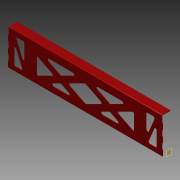
# Autodesk Inventor part: Front
Saved by Autodesk Inventor 2015 (Build 190159000, 159)
## iProperties
Created: 2014-01-06
Part Number: Front
Material: Aluminum 6061
Document SubType Name: Sheet Metal
Designer: Alex
Density: 2.71 g/cm^3
Sheet Metal Rule: Default
Appearance: Red
Author: Alex
Autodesk Inventor part; units mm, degrees
ref_plane "YZ Plane" through (0, 0, 0) normal (1, 0, 0) x (0, 1, 0)
ref_plane "XZ Plane" through (0, 0, 0) normal (0, 1, 0) x (-1, 0, 0)
ref_plane "XY Plane" through (0, 0, 0) normal (0, 0, 1) x (1, 0, 0)
sketch "Sketch1" plane through (0, 0, 0) normal (0, 0, 1) x (1, 0, 0)
  line L0 (-18.5351, 198.7023) -> (673.8689, 198.7023)
  line L1 (673.8689, 198.7023) -> (673.8689, -4.4977)
  line L2 (673.8689, -4.4977) -> (-18.5351, -4.4977)
  line L3 (-18.5351, -4.4977) -> (-18.5351, 198.7023)
  line L4 (-18.5351, 198.7023) -> (-15.9951, 198.7023)
  line L5 (-15.9951, 198.7023) -> (-15.9951, 173.3023)
  line L6 (-15.9951, 173.3023) -> (-18.5351, 173.3023)
  line L7 (-18.5351, 173.3023) -> (-18.5351, 198.7023)
  line L8 (-18.5351, -4.4977) -> (-15.9951, -4.4977)
  line L9 (-15.9951, -4.4977) -> (-15.9951, 20.9023)
  line L10 (-15.9951, 20.9023) -> (-18.5351, 20.9023)
  line L11 (-18.5351, 20.9023) -> (-18.5351, -4.4977)
  line L12 (-18.5351, 71.7023) -> (-15.9951, 71.7023)
  line L13 (-15.9951, 46.3023) -> (-18.5351, 46.3023)
  line L14 (-18.5351, 46.3023) -> (-18.5351, 71.7023)
  line L15 (-18.5351, 147.9023) -> (-15.9951, 147.9023)
  line L16 (-15.9951, 122.5023) -> (-18.5351, 122.5023)
  line L17 (-18.5351, 122.5023) -> (-18.5351, 147.9023)
  line L18 (673.8689, 198.7023) -> (671.3289, 198.7023)
  line L19 (671.3289, 198.7023) -> (671.3289, 173.3023)
  line L20 (671.3289, 173.3023) -> (673.8689, 173.3023)
  line L21 (673.8689, 173.3023) -> (673.8689, 198.7023)
  line L22 (673.8689, 147.9023) -> (671.3289, 147.9023)
  line L23 (671.3289, 122.5023) -> (673.8689, 122.5023)
  line L24 (673.8689, 122.5023) -> (673.8689, 147.9023)
  line L25 (673.8689, 71.7023) -> (671.3289, 71.7023)
  line L26 (671.3289, 46.3023) -> (673.8689, 46.3023)
  line L27 (673.8689, 46.3023) -> (673.8689, 71.7023)
  line L28 (673.8689, 20.9023) -> (671.3289, 20.9023)
  line L29 (671.3289, 20.9023) -> (671.3289, -4.4977)
  line L30 (671.3289, -4.4977) -> (673.8689, -4.4977)
  line L31 (673.8689, -4.4977) -> (673.8689, 20.9023)
  point P0 (0, 0)
  dimension "d0" = 692.404
  dimension "d1" = 203.2
  dimension "d4" = 25.4
  dimension "d6" = 25.4
  dimension "d7" = 25.4
  dimension "d8" = 25.4
  dimension "d9" = 25.4
  dimension "d10" = 25.4
  dimension "d11" = 2.54
  dimension "d12" = 25.4
  measures "d0" distance of L1.end L2.end
  measures "d1" distance between parallel lines of L2 L0
  measures "d4" distance of L4.end L5.end
  measures "d6" distance of L9.end L8.end
  measures "d7" distance of L12.end L13.start
  measures "d8" distance of L15.end L16.start
  measures "d9" distance between parallel lines of L6 L15
  measures "d10" distance between parallel lines of L10 L13
  measures "d11" distance of L20.end L19.end
  measures "d12" distance of L19.end L18.end
extrude "Plate2" add sketch "Sketch1" along normal blind 2.286 contours L0 L19 L20 L1 L28 L29 L2 L9 L10 L3 L6 L5
sketch "Sketch4" plane through (0, 0, 2.286) normal (0, 0, 1) x (1, 0, 0)
  line L0 (671.3289, 173.3023) -> (671.3289, 198.7023)
  line L1 (671.3289, 198.7023) -> (-15.9951, 198.7023)
  line L2 (-15.9951, 198.7023) -> (-15.9951, 173.3023)
  line L3 (671.3289, 20.9023) -> (-15.9951, 20.9023)
  line L4 (-15.9951, 20.9023) -> (-15.9951, -4.4977)
  line L5 (-15.9951, -4.4977) -> (671.3289, -4.4977)
  line L6 (671.3289, -4.4977) -> (671.3289, 20.9023)
  line L7 (671.3289, 173.3023) -> (671.3289, 198.7023) projected
  line L8 (-15.9951, 198.7023) -> (-15.9951, 173.3023) projected
  line L9 (-15.9951, 175.5883) -> (671.3289, 175.5883)
  line L10 (-15.9951, 198.7023) -> (671.3289, 198.7023)
  line L11 (671.3289, 198.7023) -> (671.3289, 175.5883)
  line L12 (671.3289, 175.5883) -> (-15.9951, 175.5883)
  line L13 (-15.9951, 175.5883) -> (-15.9951, 198.7023)
  point P0 (0, 0)
  constraints: 24 end point, 5 parallel, 3 perpendicular, 2 horizontal, 2 point on line
extrude "Cut1" cut sketch "Sketch4" against normal blind 2.286
sketch "Sketch12" plane through (671.3289, 177.8743, -2.286) normal (0, 1, 0) x (-1, 0, 0)
  line L0 (687.324, 0) -> (0, 0)
  line L1 (0, 0) -> (0, -33.528)
  line L2 (0, -33.528) -> (687.324, -33.528)
  line L3 (687.324, -33.528) -> (687.324, 0)
  constraints: 6 end point, 1 horizontal, 1 perpendicular, 1 vertical
edge flange "Flange6" height 38.1 angle 90 thickness 2.286 bend radius 2.286 thickness toward (0, 1, 0) relief straight relief width 2.286 relief depth 1.143 edges at (327.6669, 175.5883, 0) wall of the first edge with corners at (-15.9951, 177.8743, -2.286) (671.3289, 177.8743, -2.286) (671.3289, 177.8743, -35.814) (-15.9951, 177.8743, -35.814)
bend "Bend6"
corner "Corner6"
sketch "Sketch15" plane through (0, 0, 2.286) normal (0, 0, 1) x (1, 0, 0)
  line L0 (494.3547, 133.5854) -> (440.1051, 106.492) projected
  arc A0 (434.4307, 106.492) -> (440.1051, 106.492) centre (437.2679, 112.1729) ccw projected
  line L1 (434.4307, 106.492) -> (380.1811, 133.5854) projected
  arc A1 (383.0183, 145.6163) -> (380.1811, 133.5854) centre (383.0183, 139.2663) ccw projected
  line L2 (383.0183, 145.6163) -> (491.5175, 145.6163) projected
  arc A2 (494.3547, 133.5854) -> (491.5175, 145.6163) centre (491.5175, 139.2663) ccw projected
  line L3 (220.9031, 75.2666) -> (275.1527, 48.1732) projected
  arc A3 (272.3155, 36.1423) -> (275.1527, 48.1732) centre (272.3155, 42.4923) ccw projected
  line L4 (272.3155, 36.1423) -> (163.8163, 36.1423) projected
  arc A4 (160.9791, 48.1732) -> (163.8163, 36.1423) centre (163.8163, 42.4923) ccw projected
  line L5 (160.9791, 48.1732) -> (215.2287, 75.2666) projected
  arc A5 (220.9031, 75.2666) -> (215.2287, 75.2666) centre (218.0659, 69.5857) ccw projected
  line L6 (163.8163, 145.6163) -> (272.3155, 145.6163) projected
  arc A6 (275.1527, 133.5854) -> (272.3155, 145.6163) centre (272.3155, 139.2663) ccw projected
  line L7 (275.1527, 133.5854) -> (220.9031, 106.492) projected
  arc A7 (215.2287, 106.492) -> (220.9031, 106.492) centre (218.0659, 112.1729) ccw projected
  line L8 (215.2287, 106.492) -> (160.9791, 133.5854) projected
  arc A8 (163.8163, 145.6163) -> (160.9791, 133.5854) centre (163.8163, 139.2663) ccw projected
  line L9 (108.4649, 60.6072) -> (108.4649, 121.1514) projected
  arc A9 (117.6521, 126.8323) -> (108.4649, 121.1514) centre (114.8149, 121.1514) ccw projected
  line L10 (117.6521, 126.8323) -> (178.2665, 96.5602) projected
  arc A10 (178.2665, 85.1984) -> (178.2665, 96.5602) centre (175.4293, 90.8793) ccw projected
  line L11 (178.2665, 85.1984) -> (117.6521, 54.9263) projected
  arc A11 (108.4649, 60.6072) -> (117.6521, 54.9263) centre (114.8149, 60.6072) ccw projected
  line L12 (537.6817, 54.9263) -> (477.0674, 85.1984) projected
  arc A12 (477.0674, 96.5602) -> (477.0674, 85.1984) centre (479.9045, 90.8793) ccw projected
  line L13 (477.0674, 96.5602) -> (537.6817, 126.8323) projected
  arc A13 (546.8689, 121.1514) -> (537.6817, 126.8323) centre (540.5189, 121.1514) ccw projected
  line L14 (546.8689, 121.1514) -> (546.8689, 60.6072) projected
  arc A14 (537.6817, 54.9263) -> (546.8689, 60.6072) centre (540.5189, 60.6072) ccw projected
  line L15 (380.1811, 48.1732) -> (434.4307, 75.2666) projected
  arc A15 (440.1051, 75.2666) -> (434.4307, 75.2666) centre (437.2679, 69.5857) ccw projected
  line L16 (440.1051, 75.2666) -> (494.3547, 48.1732) projected
  arc A16 (491.5175, 36.1423) -> (494.3547, 48.1732) centre (491.5175, 42.4923) ccw projected
  line L17 (491.5175, 36.1423) -> (383.0183, 36.1423) projected
  arc A17 (380.1811, 48.1732) -> (383.0183, 36.1423) centre (383.0183, 42.4923) ccw projected
  line L18 (397.4685, 85.1984) -> (330.5041, 51.755) projected
  arc A18 (324.8297, 51.755) -> (330.5041, 51.755) centre (327.6669, 57.4359) ccw projected
  line L19 (324.8297, 51.755) -> (257.8654, 85.1984) projected
  arc A19 (257.8654, 96.5602) -> (257.8654, 85.1984) centre (260.7025, 90.8793) ccw projected
  line L20 (257.8654, 96.5602) -> (324.8297, 130.0036) projected
  arc A20 (330.5041, 130.0036) -> (324.8297, 130.0036) centre (327.6669, 124.3227) ccw projected
  line L21 (330.5041, 130.0036) -> (397.4685, 96.5602) projected
  arc A21 (397.4685, 85.1984) -> (397.4685, 96.5602) centre (394.6313, 90.8793) ccw projected
  line L22 (577.7299, 78.0523) -> (577.7299, 116.1523) projected
  arc A22 (584.0799, 122.5023) -> (577.7299, 116.1523) centre (584.0799, 116.1523) ccw projected
  line L23 (584.0799, 122.5023) -> (622.1799, 122.5023) projected
  arc A23 (628.5299, 116.1523) -> (622.1799, 122.5023) centre (622.1799, 116.1523) ccw projected
  line L24 (628.5299, 116.1523) -> (628.5299, 78.0523) projected
  arc A24 (622.1799, 71.7023) -> (628.5299, 78.0523) centre (622.1799, 78.0523) ccw projected
  line L25 (622.1799, 71.7023) -> (584.0799, 71.7023) projected
  arc A25 (577.7299, 78.0523) -> (584.0799, 71.7023) centre (584.0799, 78.0523) ccw projected
  line L26 (26.8039, 78.0523) -> (26.8039, 116.1523) projected
  arc A26 (33.1539, 122.5023) -> (26.8039, 116.1523) centre (33.1539, 116.1523) ccw projected
  line L27 (33.1539, 122.5023) -> (71.2539, 122.5023) projected
  arc A27 (77.6039, 116.1523) -> (71.2539, 122.5023) centre (71.2539, 116.1523) ccw projected
  line L28 (77.6039, 116.1523) -> (77.6039, 78.0523) projected
  arc A28 (71.2539, 71.7023) -> (77.6039, 78.0523) centre (71.2539, 78.0523) ccw projected
  line L29 (71.2539, 71.7023) -> (33.1539, 71.7023) projected
  arc A29 (26.8039, 78.0523) -> (33.1539, 71.7023) centre (33.1539, 78.0523) ccw projected
  line L30 (584.0799, 46.3023) -> (622.1799, 46.3023) projected
  arc A30 (628.5299, 39.9523) -> (622.1799, 46.3023) centre (622.1799, 39.9523) ccw projected
  line L31 (628.5299, 39.9523) -> (628.5299, 20.9023) projected
  line L32 (671.5829, 20.9023) -> (628.5299, 20.9023) projected
  line L33 (671.5829, 33.6023) -> (671.5829, 20.9023) projected
  line L34 (673.8689, 33.6023) -> (671.5829, 33.6023) projected
  line L35 (673.8689, 59.0023) -> (673.8689, 33.6023) projected
  line L36 (671.5829, 59.0023) -> (673.8689, 59.0023) projected
  line L37 (671.5829, 84.4023) -> (671.5829, 59.0023) projected
  line L38 (673.8689, 84.4023) -> (671.5829, 84.4023) projected
  line L39 (673.8689, 109.8023) -> (673.8689, 84.4023) projected
  line L40 (671.5829, 109.8023) -> (673.8689, 109.8023) projected
  line L41 (671.5829, 135.2023) -> (671.5829, 109.8023) projected
  line L42 (673.8689, 135.2023) -> (671.5829, 135.2023) projected
  line L43 (673.8689, 160.6023) -> (673.8689, 135.2023) projected
  line L44 (671.5829, 160.6023) -> (673.8689, 160.6023) projected
  line L45 (671.5829, 171.0163) -> (671.5829, 160.6023) projected
  line L46 (671.5829, 171.0163) -> (666.5029, 171.0163) projected
  line L47 (666.5029, 171.0163) -> (579.6349, 171.0163) projected
  line L48 (579.6349, 171.0163) -> (574.5549, 171.0163) projected
  line L49 (574.5549, 171.0163) -> (574.5549, 99.3883) projected
  line L50 (574.5549, 99.3883) -> (572.2689, 99.3883) projected
  line L51 (572.2689, 99.3883) -> (572.2689, 171.0163) projected
  line L52 (572.2689, 171.0163) -> (83.0649, 171.0163) projected
  line L53 (83.0649, 171.0163) -> (83.0649, 99.3883) projected
  line L54 (83.0649, 99.3883) -> (80.7789, 99.3883) projected
  line L55 (80.7789, 99.3883) -> (80.7789, 171.0163) projected
  line L56 (80.7789, 171.0163) -> (75.6989, 171.0163) projected
  line L57 (75.6989, 171.0163) -> (-11.1691, 171.0163) projected
  line L58 (-11.1691, 171.0163) -> (-16.2491, 171.0163) projected
  line L59 (-16.2491, 160.6023) -> (-16.2491, 171.0163) projected
  line L60 (-18.5351, 160.6023) -> (-16.2491, 160.6023) projected
  line L61 (-18.5351, 135.2023) -> (-18.5351, 160.6023) projected
  line L62 (-16.2491, 135.2023) -> (-18.5351, 135.2023) projected
  line L63 (-16.2491, 109.8023) -> (-16.2491, 135.2023) projected
  line L64 (-18.5351, 109.8023) -> (-16.2491, 109.8023) projected
  line L65 (-18.5351, 84.4023) -> (-18.5351, 109.8023) projected
  line L66 (-16.2491, 84.4023) -> (-18.5351, 84.4023) projected
  line L67 (-16.2491, 59.0023) -> (-16.2491, 84.4023) projected
  line L68 (-18.5351, 59.0023) -> (-16.2491, 59.0023) projected
  line L69 (-18.5351, 33.6023) -> (-18.5351, 59.0023) projected
  line L70 (-16.2491, 33.6023) -> (-18.5351, 33.6023) projected
  line L71 (-16.2491, 20.9023) -> (-16.2491, 33.6023) projected
  line L72 (26.8039, 20.9023) -> (-16.2491, 20.9023) projected
  line L73 (26.8039, 20.9023) -> (26.8039, 39.9523) projected
  arc A31 (33.1539, 46.3023) -> (26.8039, 39.9523) centre (33.1539, 39.9523) ccw projected
  line L74 (33.1539, 46.3023) -> (71.2539, 46.3023) projected
  arc A32 (77.6039, 39.9523) -> (71.2539, 46.3023) centre (71.2539, 39.9523) ccw projected
  line L75 (77.6039, 39.9523) -> (77.6039, 20.9023) projected
  line L76 (83.0649, 20.9023) -> (77.6039, 20.9023) projected
  line L77 (83.0649, 20.9023) -> (83.0649, 23.4423) projected
  line L78 (83.0649, 23.4423) -> (133.8649, 23.4423) projected
  line L79 (133.8649, 23.4423) -> (133.8649, 20.9023) projected
  line L80 (192.0944, 20.9023) -> (133.8649, 20.9023) projected
  line L81 (192.0944, 20.9023) -> (192.0944, 23.4423) projected
  line L82 (192.0944, 23.4423) -> (242.8944, 23.4423) projected
  line L83 (242.8944, 23.4423) -> (242.8944, 20.9023) projected
  line L84 (301.1239, 20.9023) -> (242.8944, 20.9023) projected
  line L85 (301.1239, 20.9023) -> (301.1239, 23.4423) projected
  line L86 (301.1239, 23.4423) -> (351.9239, 23.4423) projected
  line L87 (351.9239, 23.4423) -> (351.9239, 20.9023) projected
  line L88 (410.1533, 20.9023) -> (351.9239, 20.9023) projected
  line L89 (410.1533, 20.9023) -> (410.1533, 23.4423) projected
  line L90 (410.1533, 23.4423) -> (460.9533, 23.4423) projected
  line L91 (460.9533, 23.4423) -> (460.9533, 20.9023) projected
  line L92 (519.1828, 20.9023) -> (460.9533, 20.9023) projected
  line L93 (519.1828, 20.9023) -> (519.1828, 23.4423) projected
  line L94 (519.1828, 23.4423) -> (569.9828, 23.4423) projected
  line L95 (569.9828, 23.4423) -> (569.9828, 20.9023) projected
  line L96 (577.7299, 20.9023) -> (569.9828, 20.9023) projected
  line L97 (577.7299, 20.9023) -> (577.7299, 39.9523) projected
  arc A33 (584.0799, 46.3023) -> (577.7299, 39.9523) centre (584.0799, 39.9523) ccw projected
  line L98 (-18.5351, 20.9023) -> (673.8689, 20.9023) projected
  line L99 (380.1811, 48.1732) -> (376.9435, 46.5563)
  line L100 (494.3547, 48.1732) -> (497.5923, 46.5563)
  line L101 (275.1527, 48.1732) -> (278.3903, 46.5563)
  line L102 (160.9791, 48.1732) -> (157.7415, 46.5563)
  line L103 (157.7415, 46.5563) -> (278.3903, 46.5563)
  line L104 (376.9435, 46.5563) -> (497.5923, 46.5563)
  circle A34 centre (559.3149, 158.3163) radius 1.5875 projected
  circle A35 centre (-3.2951, 96.9031) radius 1.5875 projected
  circle A36 centre (96.0189, 158.3163) radius 1.5875 projected
  circle A37 centre (658.6289, 96.9031) radius 1.5875 projected
  circle A38 centre (327.6669, 36.3963) radius 1.5875 projected
  point P0 (0, 0)
  point P1 (373.7342, 46.3023)
  point P2 (513.5016, 46.5563)
  point P3 (281.5996, 46.3023)
  point P4 (141.8322, 46.5563)
  dimension "d139" = 25.654
  dimension "d140" = 25.654
  constraints: 12 end point, 4 tangent, 2 parallel, 2 point on line, 1 other
extrude "Cut5" cut sketch "Sketch15" against normal blind 2.286 contours L0 A0 L1 A1 L2 A2 | L3 A3 L103 A4 L5 A5 | L101 L103 A3 | A4 L103 L102 | L6 A6 L7 A7 L8 A8 | L9 A9 L10 A10 L11 A11 | L12 A12 L13 A13 L14 A14 | L15 A15 L16 A16 L104 A17 | A17 L104 L99 | A16 L100 L104 | L18 A18 L19 A19 L20 A20 L21 A21
fillet "Corner Round1" radius 6.35 4 edges at (497.5923, 46.5563, 1.143) (376.9435, 46.5563, 1.143) (157.7415, 46.5563, 1.143) (278.3903, 46.5563, 1.143)
sketch "Sketch18" plane through (0, 0, 2.286) normal (0, 0, 1) x (1, 0, 0)
  line L0 (671.3289, 175.5883) -> (-15.9951, 175.5883) projected
  line L1 (-18.5351, 147.9023) -> (-18.5351, 173.3023) projected
  line L2 (-18.5351, 20.9023) -> (673.8689, 20.9023) projected
  line L3 (673.8689, 46.3023) -> (673.8689, 20.9023) projected
  line L4 (6.8649, 156.5383) -> (55.3789, 156.5383)
  line L5 (55.3789, 156.5383) -> (55.3789, 39.9523)
  line L6 (55.3789, 39.9523) -> (6.8649, 39.9523)
  line L7 (6.8649, 39.9523) -> (6.8649, 156.5383)
  line L8 (13.7427, 156.5383) -> (55.3789, 56.4807)
  line L9 (48.5011, 39.9523) -> (6.8649, 140.0099)
  line L10 (648.4689, 156.5383) -> (599.9549, 156.5383)
  line L11 (599.9549, 156.5383) -> (599.9549, 39.9523)
  line L12 (599.9549, 39.9523) -> (648.4689, 39.9523)
  line L13 (648.4689, 39.9523) -> (648.4689, 156.5383)
  line L14 (599.9549, 56.4807) -> (641.5911, 156.5383)
  line L15 (648.4689, 140.0099) -> (606.8327, 39.9523)
  point P0 (-15.9951, 175.5883)
  point P1 (0, 0)
  point P2 (80.7789, 173.3023)
  point P3 (579.1269, 173.3023)
  point P4 (574.5549, 173.3023)
  point P5 (671.3289, 173.3023)
  point P6 (-15.9951, 173.3023)
  dimension "d169" = 19.05
  dimension "d170" = 25.4
  dimension "d171" = 19.05
  dimension "d172" = 25.4
  dimension "d173" = 12.7
  dimension "d174" = 6.35
  dimension "d175" = 6.35
  dimension "d176" = 19.05
  dimension "d177" = 25.4
  dimension "d178" = 19.05
  dimension "d180" = 6.35
  dimension "d181" = 6.35
  dimension "d182" = 12.7
  dimension "d186" = 25.4
  constraints: 24 end point, 8 point on line, 6 parallel, 2 horizontal, 2 perpendicular, 4 other
  measures "d170" distance between parallel lines of L1 L7
  measures "d171" distance between parallel lines of L2 L6
  measures "d172" distance from line of L5 point (80.779, 173.302)
  measures "d173" distance between parallel lines of L9 L8
  measures "d174" distance from line of L4.start L8
  measures "d175" distance from line of L5.end L9
  measures "d176" distance between parallel lines of L2 L12
  measures "d177" distance between parallel lines of L3 L13
  measures "d180" distance from line of L10.start L14
  measures "d181" distance from line of L11.end L15
  measures "d182" distance between parallel lines of L14 L15
  measures "d186" distance from line of point (574.555, 173.302) L11
extrude "Cut7" cut sketch "Sketch18" against normal blind 2.286 contours L4 L5 L8 | L9 L6 L7 | L14 L11 L10 | L13 L12 L15
fillet "Corner Round3" radius 6.35 12 edges at (13.7427, 156.5383, 1.143) (55.3789, 56.4807, 1.143) (48.5011, 39.9523, 1.143) (6.8649, 39.9523, 1.143) (6.8649, 140.0099, 1.143) (55.3789, 156.5383, 1.143) (599.9549, 56.4807, 1.143) (606.8327, 39.9523, 1.143) (648.4689, 39.9523, 1.143) (641.5911, 156.5383, 1.143) (648.4689, 140.0099, 1.143) (599.9549, 156.5383, 1.143)
sketch "Sketch19" plane through (0, 0, 2.286) normal (0, 0, 1) x (1, 0, 0)
  line L0 (-15.9951, 175.5883) -> (-13.4551, 175.5883)
  line L1 (-13.4551, 175.5883) -> (-13.4551, 174.3183)
  line L2 (-13.4551, 174.3183) -> (-15.9951, 174.3183)
  line L3 (-15.9951, 174.3183) -> (-15.9951, 175.5883)
  line L4 (671.3289, 175.5883) -> (668.7889, 175.5883)
  line L5 (668.7889, 175.5883) -> (668.7889, 174.3183)
  line L6 (668.7889, 174.3183) -> (671.3289, 174.3183)
  line L7 (671.3289, 174.3183) -> (671.3289, 175.5883)
  line L8 (-15.9951, 175.5883) -> (-13.4551, 175.5883)
  line L9 (-13.4551, 175.5883) -> (-13.4551, 174.3183)
  line L10 (-13.4551, 174.3183) -> (-15.9951, 174.3183)
  line L11 (-15.9951, 174.3183) -> (-15.9951, 175.5883)
  line L12 (-13.4551, 174.3183) -> (-15.9951, 174.3183)
  line L13 (-15.9951, 174.3183) -> (-15.9951, 175.5883)
  line L14 (-15.9951, 175.5883) -> (-13.4551, 175.5883)
  line L15 (-13.4551, 175.5883) -> (-13.4551, 174.3183)
  point P0 (0, 0)
  dimension "d187" = 2.54
  dimension "d188" = 1.27
  dimension "d189" = 2.54
  dimension "d190" = 1.27
  constraints: 32 end point, 8 parallel, 4 horizontal, 4 perpendicular
  measures "d187" distance of L1.end L2.end
  measures "d188" distance of L0.end L1.end
  measures "d189" distance of L6.end L5.end
  measures "d190" distance of L5.end L4.end
extrude "Cut8" cut sketch "Sketch19" against normal blind 2.286
ref_plane "Work Plane1" through (678.4409, 20.9023, -23.114) normal (1, 0, 0) x (0, 0, -1)
sketch "Sketch20" plane through (678.4409, 20.9023, -23.114) normal (1, 0, 0) x (0, 0, -1)
  circle A0 centre (-10.414, 127) radius 1.7907
  circle A1 centre (-10.414, 127) radius 1.7907
  circle A2 centre (-10.414, 127) radius 1.7907 projected
  point P0 (-23.114, -20.9023)
  dimension "d213" = 3.5814
  constraints: 2 centre point, 2 concentric, 1 coincident
  measures "d213" diameter of A0
extrude "Cut9" cut sketch "Sketch20" along normal through all both and the other way through all
sketch "Sketch21" plane through (0, 0, 2.286) normal (0, 0, 1) x (1, 0, 0)
  line L0 (500.652, 25.4743) -> (155.4152, 25.4743) projected
  line L1 (155.4152, 46.3023) -> (155.4152, 25.4743) projected
  line L2 (155.4152, 46.3023) -> (500.652, 46.3023) projected
  line L3 (500.652, 46.3023) -> (500.652, 25.4743) projected
  circle A0 centre (206.2152, 35.8883) radius 1.5875
  circle A1 centre (449.852, 35.8883) radius 1.5875
  circle A2 centre (206.2152, 35.8883) radius 1.5875 projected
  circle A3 centre (449.852, 35.8883) radius 1.5875 projected
  point P0 (0, 0)
  dimension "d199" = 3.175
  dimension "d200" = 10.414
  dimension "d201" = 10.414
  dimension "d202" = 50.8
  dimension "d203" = 10.414
  dimension "d204" = 50.8
  constraints: 2 centre point
  measures "d199" diameter of A0
  measures "d200" distance from line of L0 A0.centre
  measures "d201" distance from line of L2 A0.centre
  measures "d202" distance from line of L1 A0.centre
  measures "d203" distance from line of L0 A1.centre
  measures "d204" distance from line of L3 A1.centre
extrude "Cut10" cut sketch "Sketch21" against normal blind 2.286 contours A0 | A1
sketch "Sketch22" plane through (0, 0, 2.286) normal (0, 0, 1) x (1, 0, 0)
  line L0 (576.8409, 173.3023) -> (576.8409, 20.9023) projected
  line L1 (597.6689, 20.9023) -> (576.8409, 20.9023) projected
  line L2 (597.6689, 173.3023) -> (597.6689, 20.9023) projected
  line L3 (78.4929, 173.3023) -> (78.4929, 20.9023) projected
  line L4 (57.6649, 20.9023) -> (78.4929, 20.9023) projected
  line L5 (57.6649, 20.9023) -> (57.6649, 173.3023) projected
  circle A0 centre (68.0789, 71.7023) radius 1.5875 projected
  line L6 (57.6649, 173.3023) -> (78.4929, 173.3023) projected
  circle A1 centre (587.2549, 71.7023) radius 1.5875 projected
  line L7 (576.8409, 173.3023) -> (597.6689, 173.3023) projected
  circle A2 centre (68.0789, 71.7023) radius 1.5875
  circle A3 centre (587.2549, 71.7023) radius 1.5875
  point P0 (0, 0)
  constraints: 2 centre point, 2 coincident, 2 concentric
extrude "Cut11" cut sketch "Sketch22" against normal blind 2.286 contours A0 | A1
sketch "Sketch26" plane through (0, 0, 2.286) normal (0, 0, 1) x (1, 0, 0)
  line L0 (-15.9951, 173.3023) -> (-18.5351, 173.3023) projected
  line L1 (-18.5351, 20.9023) -> (-18.5351, 173.3023) projected
  line L2 (673.8689, 173.3023) -> (673.8689, 20.9023) projected
  line L3 (673.8689, 173.3023) -> (671.3289, 173.3023) projected
  line L4 (673.8689, 147.9023) -> (671.5829, 147.9023)
  line L5 (671.5829, 173.3023) -> (671.5829, 147.9023)
  line L6 (673.8689, 173.3023) -> (671.5829, 173.3023)
  line L7 (673.8689, 173.3023) -> (673.8689, 147.9023)
  line L8 (673.8689, 97.1023) -> (671.5829, 97.1023)
  line L9 (671.5829, 122.5023) -> (671.5829, 97.1023)
  line L10 (673.8689, 122.5023) -> (671.5829, 122.5023)
  line L11 (673.8689, 122.5023) -> (673.8689, 97.1023)
  line L12 (673.8689, 46.3023) -> (671.5829, 46.3023)
  line L13 (671.5829, 71.7023) -> (671.5829, 46.3023)
  line L14 (673.8689, 71.7023) -> (671.5829, 71.7023)
  line L15 (673.8689, 71.7023) -> (673.8689, 46.3023)
  line L16 (-16.2491, 147.9023) -> (-16.2491, 173.3023)
  line L17 (-18.5351, 147.9023) -> (-16.2491, 147.9023)
  line L18 (-16.2491, 147.9023) -> (-18.5351, 147.9023)
  line L19 (-18.5351, 147.9023) -> (-18.5351, 173.3023)
  line L20 (-18.5351, 173.3023) -> (-16.2491, 173.3023)
  line L21 (-16.2491, 173.3023) -> (-16.2491, 147.9023)
  line L22 (-18.5351, 97.1023) -> (-16.2491, 97.1023)
  line L23 (-18.5351, 97.1023) -> (-18.5351, 122.5023)
  line L24 (-18.5351, 122.5023) -> (-16.2491, 122.5023)
  line L25 (-16.2491, 122.5023) -> (-16.2491, 97.1023)
  line L26 (-18.5351, 46.3023) -> (-16.2491, 46.3023)
  line L27 (-18.5351, 46.3023) -> (-18.5351, 71.7023)
  line L28 (-18.5351, 71.7023) -> (-16.2491, 71.7023)
  line L29 (-16.2491, 71.7023) -> (-16.2491, 46.3023)
  line L30 (-18.5351, 122.5023) -> (-16.2491, 122.5023)
  line L31 (-16.2491, 122.5023) -> (-16.2491, 97.1023)
  line L32 (-16.2491, 97.1023) -> (-18.5351, 97.1023)
  line L33 (-18.5351, 97.1023) -> (-18.5351, 122.5023)
  line L34 (-18.5351, 71.7023) -> (-16.2491, 71.7023)
  line L35 (-16.2491, 71.7023) -> (-16.2491, 46.3023)
  line L36 (-16.2491, 46.3023) -> (-18.5351, 46.3023)
  line L37 (-18.5351, 46.3023) -> (-18.5351, 71.7023)
  point P0 (0, 0)
  dimension "d216" = 50.8
  dimension "d223" = 50.8
  constraints: 68 end point, 6 horizontal, 6 parallel, 5 vertical, 3 perpendicular, 41 other
  measures "d216" distance of L5.start L9.start
  measures "d223" distance of L0.end L24.start
extrude "Cut13" cut sketch "Sketch26" against normal blind 2.286
equation "\"d26\" = Thickness"
equation "\"d88\" = BendReliefWidth"
equation "\"d89\" = BendReliefDepth"
equation "\"d90\" = MinimumRemnant"
equation "\"d91\" = BendRadius"
equation "\"d94\" = BendRadius"
equation "\"d95\" = CornerReliefSize"
equation "\"d96\" = GapSize"
equation "\"d97\" = JacobiRadiusSize"
equation "\"BendRadius\" = Thickness"
equation "\"BendReliefWidth\" = Thickness"
equation "\"BendReliefDepth\" = 0.5 * Thickness"
equation "\"CornerReliefSize\" = 4 * Thickness"
equation "\"MinimumRemnant\" = 2 * Thickness"
equation "\"TransitionRadius\" = BendRadius"
equation "\"JacobiRadiusSize\" = BendRadius"
equation "\"GapSize\" = Thickness"
equation "\"d2\" = BendRadius"
equation "\"d13\" = BendRadius"
equation "\"Thickness\" = 2.286"
body "Solid2"
